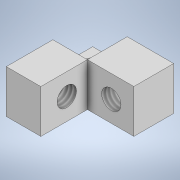
# Autodesk Inventor part: fileholddub
Saved by Autodesk Inventor 2020 (Build 240168000, 168)
## iProperties
Created: 2019-06-14
Part Number: fileholddub
Material: Generic
Document SubType Name: Modeling
Designer: ColinP
Density: 1 g/cm^3
Appearance: Default
Mass: 0.443713 g
Surface Area: 6.08545 cm^2
Volume: 0.443713 cm^3
Author: ColinP
Autodesk Inventor part; units mm, degrees
ref_plane "YZ Plane" through (0, 0, 0) normal (1, 0, 0) x (0, 1, 0)
ref_plane "XZ Plane" through (0, 0, 0) normal (0, 1, 0) x (-1, 0, 0)
ref_plane "XY Plane" through (0, 0, 0) normal (0, 0, 1) x (1, 0, 0)
sketch "Sketch20" plane through (0, 0, 0) normal (0, 1, 0) x (-1, 0, 0)
  line L0 (1.5185, -0.8925) -> (-3.5615, -0.8925)
  line L1 (-3.5615, -0.8925) -> (-3.5615, 11.8075)
  line L2 (-3.5615, 11.8075) -> (1.5185, 11.8075)
  line L3 (1.5185, 11.8075) -> (1.5185, -0.8925)
  line L4 (1.5185, 4.9634) -> (-3.5615, 4.9634)
  point P0 (0, 0)
  dimension "d56" = 5.08
  dimension "d57" = 12.7
  constraints: 10 end point, 2 parallel, 2 perpendicular, 2 point on line, 1 horizontal
  measures "d56" distance of L1.end L2.end
  measures "d57" distance of L0.end L1.end
extrude "Extrusion7" add sketch "Sketch20" along normal blind 2.54 contours L0 L1 L4 L3
extrude "Extrusion8" add sketch "Sketch20" along normal blind 6.35 contours L4 L1 L2 L3
sketch "Sketch21" plane through (0, 2.54, 0) normal (0, 1, 0) x (1, 0, 0)
  line L0 (3.5615, 0.8925) -> (-1.5185, 0.8925) projected
  line L1 (-1.5185, 0.8925) -> (-1.5185, -4.9634) projected
  point P0 (0, 0)
  point P1 (1.0215, -1.6475)
  dimension "d62" = 2.54
  dimension "d63" = 2.54
  measures "d62" distance from line of L0 point (1.021, -1.648)
  measures "d63" distance from line of L1 point (1.021, -1.648)
hole "Hole5" at (1.0215, 2.54, 1.6475) direction (0, -1, 0) diameter 3.175 end through all
sketch "Sketch22" plane through (3.5615, 0, -0.8925) normal (1, 0, 0) x (0, 0, -1)
  line L0 (-12.7, 6.35) -> (-5.8558, 6.35) projected
  line L1 (-12.7, 0) -> (-12.7, 6.35) projected
  point P0 (-0.8925, 0)
  point P1 (-8.89, 3.175)
  dimension "d71" = 3.175
  dimension "d72" = 3.81
  measures "d71" distance from line of L0 point (-8.89, 3.175)
  measures "d72" distance from line of L1 point (-8.89, 3.175)
hole "Hole6" at (3.5615, 3.175, 7.9975) direction (-1, 0, 0) diameter 2.85 end through all thread size "M3.5x0.6" class "6H" standard "ISO Metric profile"
sketch "Sketch23" plane through (3.5615, 0, -0.8925) normal (1, 0, 0) x (0, 0, -1)
  line L0 (-5.8558, 2.54) -> (-5.8558, 6.35) projected
  line L1 (-5.8558, 2.54) -> (-5.8558, 0)
  line L2 (-12.7, 0) -> (0, 0) projected
  line L3 (-5.8558, 2.54) -> (0, 2.54) projected
  line L4 (-5.8558, 2.54) -> (0, 2.54)
  line L5 (0, 2.54) -> (0, 0)
  point P0 (-0.8925, 0)
  constraints: 6 end point, 1 collinear, 1 perpendicular, 1 point on line, 1 vertical
extrude "Extrusion9" add sketch "Sketch23" along normal blind 6.8326
sketch "Sketch24" plane through (0, 2.54, 0) normal (0, 1, 0) x (1, 0, 0)
  line L0 (3.5615, -4.9634) -> (10.3941, -4.9634) projected
  line L1 (3.5615, -4.9634) -> (3.5615, 0.8925)
  line L2 (-1.5185, 0.8925) -> (10.3941, 0.8925) projected
  line L3 (3.5615, 0.8925) -> (10.3941, 0.8925)
  line L4 (3.5615, -11.8075) -> (3.5615, -4.9634) projected
  line L5 (10.3941, -4.9634) -> (3.5615, -4.9634)
  line L6 (3.5615, -4.9634) -> (10.4876, -4.9634)
  line L7 (10.4876, -4.9634) -> (10.3941, -4.9634)
  line L8 (10.3941, -4.9634) -> (10.3941, 0.807)
  line L9 (10.3941, 0.807) -> (10.3941, 0.8925)
  point P0 (0, 0)
  constraints: 14 end point, 2 collinear, 2 horizontal, 2 point on line, 1 perpendicular, 1 vertical
extrude "Extrusion10" add sketch "Sketch24" along normal blind 3.81
sketch "Sketch25" plane through (-1.5185, 0, -0.8925) normal (0, 0, -1) x (-1, 0, 0)
  line L0 (-11.9126, 6.35) -> (-5.08, 6.35) projected
  line L1 (-11.9126, 0) -> (-11.9126, 6.35) projected
  point P0 (-1.5185, 0)
  point P1 (-8.5968, 3.06)
  dimension "d84" = 3.29
  dimension "d85" = 3.3158
  measures "d84" distance from line of L0 point (-8.597, 3.06)
  measures "d85" distance from line of L1 point (-8.597, 3.06)
hole "Hole7" at (7.0783, 3.06, -0.8925) direction (0, 0, 1) diameter 2.85 end through all thread size "M3.5x0.6" class "6H" standard "ISO Metric profile"
body "Solid2"
